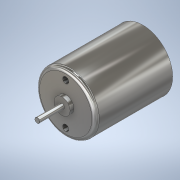
# Autodesk Inventor part: tamiya_sporttuned
Saved by Autodesk Inventor 2020 (Build 240168000, 168)
## iProperties
Created: 2021-06-14
Part Number: tamiya_sporttuned
Material: 一般
Document SubType Name: Modeling
Designer: fmasa
Density: 1 g/cm^3
Appearance: クロム - つや出し
Author: fmasa
Autodesk Inventor part; units mm, degrees
ref_plane "YZ Plane" through (0, 0, 0) normal (1, 0, 0) x (0, 1, 0)
ref_plane "XZ Plane" through (0, 0, 0) normal (0, 1, 0) x (-1, 0, 0)
ref_plane "XY Plane" through (0, 0, 0) normal (0, 0, 1) x (1, 0, 0)
sketch "スケッチ1" plane through (0, 0, 0) normal (0, 0, 1) x (1, 0, 0)
  circle A0 centre (0, 0) radius 12
  dimension "d0" = 24
  constraints: 1 centre point, 1 coincident
  measures "d0" diameter of A0
extrude "押し出し1" add sketch "スケッチ1" along normal blind 31
sketch "スケッチ2" plane through (0, 0, 31) normal (0, 0, 1) x (1, 0, 0)
  circle A0 centre (0, 0) radius 9.8 construction
  line L0 (0, -16.8) -> (0, 16.8) construction
  circle A1 centre (0, 8.3) radius 1.5
  circle A2 centre (0, -8.3) radius 1.5
  circle A3 centre (0, 0) radius 3.25
  dimension "d3" = 19.6
  dimension "d4" = 3
  dimension "d5" = 3
  dimension "d6" = 6.5
  constraints: 4 centre point, 2 coincident, 2 point on line, 2 tangent
  measures "d3" diameter of A0
  measures "d4" diameter of A1
  measures "d5" diameter of A2
  measures "d6" diameter of A3
extrude "押し出し2" add sketch "スケッチ2" along normal blind 1.5 contours A3
hole "穴1" at (0, 8.3, 31) at (0, -8.3, 31) direction (0, 0, -1) diameter 2.459 depth 8.8 tip angle 118 thread size "M3x0.5" class "6H" standard "ANSI Metric M Profile"
fillet "フィレット1" radius 1.5 1 edges at (-12, 0, 31)
sketch "スケッチ3" plane through (0, 0, 32.5) normal (0, 0, 1) x (1, 0, 0)
  circle A0 centre (0, 0) radius 3.25 projected
  circle A1 centre (0, 0) radius 1
  dimension "d17" = 2
  constraints: 1 centre point, 1 coincident
  measures "d17" diameter of A1
extrude "押し出し3" add sketch "スケッチ3" along normal blind 10 contours A1
fillet "フィレット2" radius 0.1 1 edges at (-1, 0, 42.5)
